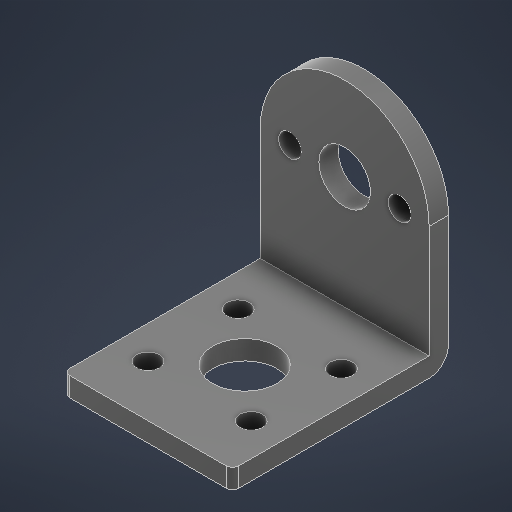
# Autodesk Inventor part: suporte
Saved by Autodesk Inventor 2026 (Build 300175000, 175)
## iProperties
Created: 2025-04-15
Part Number: suporte
Material: Generic
Document SubType Name: Modeling
Designer: ADM
Density: 1 g/cm^3
Appearance: Smooth - Black
Author: ADM
Autodesk Inventor part; units mm, degrees
ref_plane "YZ Plane" through (0, 0, 0) normal (1, 0, 0) x (0, 1, 0)
ref_plane "XZ Plane" through (0, 0, 0) normal (0, 1, 0) x (-1, 0, 0)
ref_plane "XY Plane" through (0, 0, 0) normal (0, 0, 1) x (1, 0, 0)
sketch "Sketch1" plane through (0, 0, 0) normal (0, 1, 0) x (-1, 0, 0)
  line L0 (0, 0) -> (26.2, 0)
  line L1 (26.2, 0) -> (26.2, -33.5)
  line L2 (26.2, -33.5) -> (0, -33.5)
  line L3 (0, -33.5) -> (0, 0)
  dimension "d0" = 26.2
  dimension "d1" = 33.5
  constraints: 8 end point, 2 parallel, 1 horizontal, 1 perpendicular
  measures "d0" distance of L1.end L2.end
  measures "d1" distance of L0.end L1.end
extrude "Extrusion1" add sketch "Sketch1" along normal blind 3
sketch "Sketch2" plane through (0, 3, 0) normal (0, 1, 0) x (1, 0, 0)
  line L0 (0, 33.5) -> (-26.2, 33.5) projected
  line L1 (-26.2, 33.5) -> (0, 33.5)
  line L2 (0, 33.5) -> (0, 30.5)
  line L3 (0, 30.5) -> (-26.2, 30.5)
  line L4 (-26.2, 30.5) -> (-26.2, 33.5)
  point P0 (0, 0)
  dimension "d4" = 26.2
  dimension "d5" = 3
  constraints: 8 end point, 2 parallel, 1 horizontal, 1 perpendicular
  measures "d4" distance of L2.end L3.end
  measures "d5" distance of L1.end L2.end
extrude "Extrusion2" add sketch "Sketch2" along normal blind 30.5
fillet "Fillet1" radius 3 1 edges at (-13.1, 0, -33.5)
fillet "Fillet2" radius 13.1 2 edges at (0, 33.5, -32) (-26.2, 33.5, -32)
fillet "Fillet3" radius 1 2 edges at (-26.2, 1.5, 0) (0, 1.5, 0)
sketch "Sketch3" plane through (0, 3, 0) normal (0, 1, 0) x (1, 0, 0)
  circle A0 centre (-13.1, 15) radius 5
  line L0 (0, 1) -> (0, 30.5) projected
  line L1 (-25.2, 0) -> (-1, 0) projected
  circle A1 centre (-21.1, 8) radius 1.75
  line L2 (-26.2, 30.5) -> (-26.2, 1) projected
  circle A2 centre (-5.1, 8) radius 1.75
  circle A3 centre (-21.1, 22) radius 1.75
  circle A4 centre (-5.1, 22) radius 1.75
  point P0 (0, 0)
  dimension "d11" = 10
  dimension "d12" = 13.1
  dimension "d13" = 15
  dimension "d14" = 3.5
  dimension "d15" = 7
  dimension "d16" = 5.1
  dimension "d19" = 16
  dimension "d22" = 14
  constraints: 5 centre point, 1 horizontal, 1 vertical, 6 other
  measures "d11" diameter of A0
  measures "d12" distance from line of L0 A0.centre
  measures "d13" distance from line of L1 A0.centre
  measures "d14" diameter of A1
  measures "d15" vertical distance of A0.centre A1.centre
  measures "d16" distance from line of L2 A1.centre
  measures "d19" distance of A1.centre A2.centre
  measures "d22" distance of A1.centre A3.centre
extrude "Extrusion3" cut sketch "Sketch3" against normal through all
sketch "Sketch4" plane through (0, 3, -33.5) normal (0, 0, -1) x (-1, 0, 0)
  circle A0 centre (13.1, 17.5) radius 4
  arc A1 (26.2, 17.4) -> (0, 17.4) centre (13.1, 17.4) ccw projected
  line L0 (0, 0) -> (0, 17.4) projected
  circle A2 centre (4.6, 17.5) radius 1.75
  circle A3 centre (21.6, 17.5) radius 1.75
  point P0 (0, -3)
  point P1 (13.1, 30.5)
  dimension "d27" = 8
  dimension "d28" = 13
  dimension "d32" = 13.1
  dimension "d33" = 3.5
  dimension "d34" = 4.6
  dimension "d35" = 3.5
  dimension "d36" = 17
  constraints: 3 centre point, 1 point on circle
  measures "d27" diameter of A0
  measures "d28" distance of A0.centre point (13.1, 30.5)
  measures "d32" distance from line of L0 A0.centre
  measures "d33" diameter of A2
  measures "d34" distance from line of L0 A2.centre
  measures "d35" diameter of A3
  measures "d36" distance of A3.centre A2.centre
extrude "Extrusion4" cut sketch "Sketch4" against normal through all
body "Solid1"
